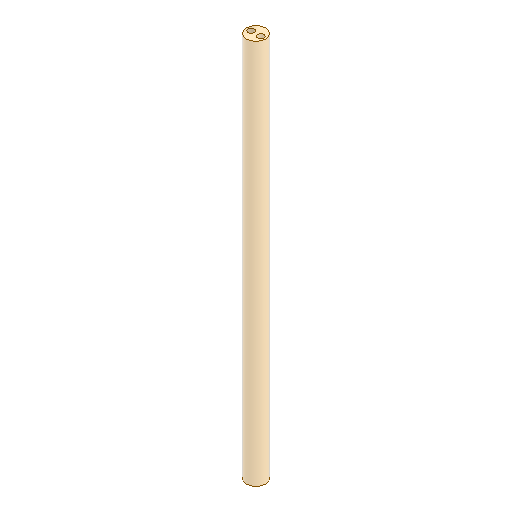
# Autodesk Inventor part: ceramic_2-hole-spacer_d3
Saved by Autodesk Inventor 2026.2 (Build 302298000, 298)
## iProperties
Created: 2026-05-08
Part Number: ceramic_2-hole-spacer_d3
Material: Generic
Document SubType Name: Modeling
Designer: zetsu
Density: 1 g/cm^3
Appearance: 滑らか - オフホワイト
Author: zetsu
Autodesk Inventor part; units mm, degrees
ref_plane "YZ Plane" through (0, 0, 0) normal (1, 0, 0) x (0, 1, 0)
ref_plane "XZ Plane" through (0, 0, 0) normal (0, 1, 0) x (-1, 0, 0)
ref_plane "XY Plane" through (0, 0, 0) normal (0, 0, 1) x (1, 0, 0)
sketch "スケッチ2" plane through (0, 0, 0) normal (0, 1, 0) x (-1, 0, 0)
  circle A0 centre (0, 0) radius 1.5
  circle A1 centre (0.75, 0) radius 0.5
  circle A2 centre (-0.75, 0) radius 0.5
  line L0 (0, 0) -> (0, -2.3561) construction
  dimension "d7" = 3
  dimension "d8" = 1
  dimension "d9" = 1
  dimension "d11" = 1.5
  constraints: 3 centre point, 2 end point, 1 coincident, 1 symmetric about line, 1 vertical
  measures "d7" diameter of A0
  measures "d8" diameter of A1
  measures "d9" diameter of A2
  measures "d11" distance of A2.centre A1.centre
extrude "押し出し2" add sketch "スケッチ2" along normal blind 60
